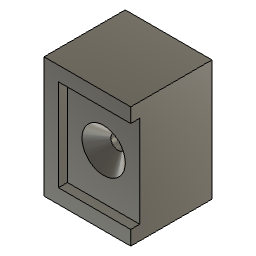
model (Autodesk Fusion 360 design; units mm, degrees)
Autodesk Fusion 360 part; units mm, degrees
sketch "Sketch1" plane through (0, 0, 0) normal (1, 0, 0) x (0, 1, 0)
  line L0 (0, 0) -> (22.5, 0)
  line L1 (22.5, 0) -> (22.5, 33.4)
  line L2 (22.5, 33.4) -> (0, 33.4)
  line L3 (0, 33.4) -> (0, 29.4)
  line L4 (0, 29.4) -> (2.5, 29.4)
  line L5 (0, 0) -> (0, 4)
  line L6 (0, 4) -> (2.5, 4)
  line L7 (2.5, 29.4) -> (2.5, 4)
  line L8 (2.5, 29.4) -> (2.5, 33.4) construction
  line L9 (0, 29.4) -> (0, 4)
  dimension "d1" = 25.4
  dimension "d4" = 4
  dimension "d5" = 2.5
  dimension "d6" = 20
  constraint horizontal L0
  constraint vertical L1
  constraint horizontal L2
  constraint vertical L3
  constraint horizontal L4
  constraint vertical L5
  constraint horizontal L6
  constraint vertical L7
  constraint equal L4 L6
  constraint equal L3 L5
  constraint coincident L0.start L5.start
  constraint coincident L2 L8.end
  constraint vertical L8
  measures "d1" distance of L3.end L5.end
  measures "d4" distance of L2.end L3.end
  measures "d5" distance of L2.end L8.end
  measures "d6" distance of L1.end L8.end
extrude "Extrude1" add sketch "Sketch1" along normal blind 20 contours L0 L1 L2 L3 L4 L5 L6 L7
extrude "Extrude2" add sketch "Sketch1" against normal blind 4
sketch "Sketch2" plane through (0, 2.5, 0) normal (0, -1, 0) x (1, 0, 0)
  line L0 (0, 29.4) -> (0, 4)
  line L1 (0, 4) -> (20, 4)
  line L2 (20, 4) -> (20, 29.4)
  line L3 (20, 29.4) -> (0, 29.4)
  circle A0 centre (10, 16.7) radius 2
  line L4 (10, 16.7) -> (10, 29.4) construction
  line L5 (10, 16.7) -> (0, 16.7) construction
  dimension "d11" = 4
  constraint coincident A0.centre L4.start
  constraint midpoint L3 L4.end
  constraint midpoint L0 L5.end
  constraint horizontal L5
  constraint vertical L4
  measures "d11" diameter of A0
extrude "Extrude3" cut sketch "Sketch2" against normal up to surface (20 mm away) contours A0
chamfer "Chamfer1" distance 4 angle 45 1 edges at (8.1353, 2.5, 17.4232)
equation "d1 = 1\""
named bodies: "alu-bracket"
